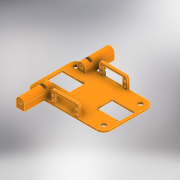
# Autodesk Inventor part: Base
Saved by Autodesk Inventor 2021 (Build 250183000, 183)
## iProperties
Created: 2024-04-05
Part Number: Base
Material: PLA
Document SubType Name: Modeling
Designer: Martin
Density: 1.27 g/cm^3
Appearance: PLA
Mass: 116.332 g
Surface Area: 562.833 cm^2
Volume: 116.332 cm^3
Author: Martin
Autodesk Inventor part; units mm, degrees
ref_plane "YZ Plane" through (0, 0, 0) normal (1, 0, 0) x (0, 1, 0)
ref_plane "XZ Plane" through (0, 0, 0) normal (0, 1, 0) x (-1, 0, 0)
sketch "Sketch1" plane through (0, 0, 0) normal (0, 0, 1) x (1, 0, 0)
  line L0 (-20.5, 0.0342) -> (20.5, 0.0342)
  line L1 (20.5, 0.0342) -> (20.5, 21.0342)
  line L2 (20.5, 21.0342) -> (-20.5, 21.0342)
  line L3 (-20.5, 21.0342) -> (-20.5, 0.0342)
  line L4 (0, -10.9658) -> (0, 38.0342) projected
  line L5 (20.5, 0.0342) -> (27.5, 0.0342)
  line L6 (20.5, 18.3469) -> (20.5, 0.0342)
  line L7 (20.5, 1.1342) -> (27.5, 1.1342)
  line L8 (27.5, 1.1342) -> (27.5, 19.9342)
  line L9 (27.5, 19.9342) -> (20.5, 19.9342)
  line L10 (20.5, 19.9342) -> (20.5, 1.1342)
  circle A0 centre (25.8, 15.5342) radius 2.3
  circle A1 centre (25.8, 5.5342) radius 2.3
  line L11 (-20.5, 0.0342) -> (-27.5, 0.0342)
  line L12 (-20.5, 1.1342) -> (-27.5, 1.1342)
  line L13 (-27.5, 19.9342) -> (-20.5, 19.9342)
  circle A2 centre (-25.8, 15.5342) radius 2.3
  circle A3 centre (-25.8, 5.5342) radius 2.3
  line L14 (-30.5, 0.0342) -> (-30.5, 31.0342)
  line L15 (30.5, 31.0342) -> (30.5, 0.0342)
  line L16 (-30.5, 26.0342) -> (30.5, 26.0342)
  line L17 (-27.5, 1.1342) -> (-27.5, 13.985)
  line L18 (-27.5, 17.0834) -> (-27.5, 19.9342)
  line L19 (-20.5, 8.5342) -> (-22.5, 8.5342)
  line L20 (-22.5, 8.5342) -> (-22.5, 12.5342)
  line L21 (-22.5, 12.5342) -> (-20.5, 12.5342)
  line L22 (-20.5, 9.5596) -> (-20.5, 7.5596)
  line L23 (-21.9602, 10.5342) -> (-18.6691, 10.5342)
  line L24 (-30.5, 0.0342) -> (-26.5, 0.0342)
  line L25 (-30.5, 0.0342) -> (30.5, 0.0342)
  line L26 (30.5, 0.0342) -> (30.5, -3.9658)
  line L27 (30.5, -3.9658) -> (-30.5, -3.9658)
  line L28 (-30.5, -3.9658) -> (-30.5, 0.0342)
  point P0 (0, 0)
  point P1 (30.5, 0.0342)
  dimension "d0" = 41
  dimension "d4" = 7
  dimension "d5" = 18.8
  dimension "d6" = 1.1
  dimension "d7" = 21
  dimension "d8" = 4.6
  dimension "d9" = 4.6
  dimension "d10" = 5.3
  dimension "d11" = 10
  dimension "d12" = 4.4
  dimension "d13" = 4.4
  dimension "d14" = 10
  dimension "d15" = 5
  dimension "d16" = 2
  dimension "d17" = 4
  dimension "d19" = 4
  constraints: 56 end point, 9 parallel, 7 horizontal, 7 symmetric about line, 4 centre point, 4 perpendicular, 3 point on line, 2 point on circle, 1 vertical alignment, 4 other
  measures "d0" distance of L0.start L0.end
  measures "d4" distance of L9.end L8.end
  measures "d5" distance of L8.end L7.end
  measures "d6" distance between parallel lines of L5 L7
  measures "d7" distance of L2.end L0.start
  measures "d8" diameter of A0
  measures "d9" diameter of A1
  measures "d10" distance from line of L6 A1.centre
  measures "d11" distance of A0.centre A1.centre
  measures "d12" distance from line of L9 A0.centre
  measures "d13" distance from line of L7 A1.centre
  measures "d14" distance between parallel lines of L3 L14
  measures "d15" distance between parallel lines of L2 L16
  measures "d16" distance of L20.end L21.end
  measures "d17" distance of L19.end L20.end
  measures "d19" distance of L25.end L26.end
extrude "Extrusion1" add sketch "Sketch1" along normal blind 5 contours L11 L24 L14 L16 L4 L2 L3 L13 L18 A2 L17 A3 L12 | L0 L4 L27 L28 L24 L11 | L0 L5 L25 L26 L27 L4 | L12 L17 A3 A2 L18 L13 L3 L21 L20 L19 | L1 L7 L8 A1 A0 L9 L2 L4 L16 L15 L25 L5 | L1 L9 L8 A0 A1 L7
sketch "Sketch2" plane through (0, 0, 5) normal (0, 0, 1) x (1, 0, 0)
  line L0 (20.5, 0.0342) -> (-20.5, 0.0342) projected
  line L1 (20.5, 0.0342) -> (12.9, 0.0342)
  line L2 (12.9, 0.0342) -> (12.9, 10.0342)
  line L3 (12.9, 10.0342) -> (-54.1, 10.0342)
  circle A0 centre (-54.1, 10.0342) radius 4.1
  circle A1 centre (-54.1, 10.0342) radius 9.1
  line L4 (-63.2, 10.0342) -> (-63.2, 0.0342)
  line L5 (-45, 10.0342) -> (-45, 0.0342)
  line L6 (-63.2, 0.0342) -> (-45, 0.0342)
  line L7 (-63.2, 0.0342) -> (-45, 0.0342)
  line L8 (-45, 0.0342) -> (-45, -3.9658)
  line L9 (-45, -3.9658) -> (-63.2, -3.9658)
  line L10 (-63.2, -3.9658) -> (-63.2, 0.0342)
  point P0 (0, 0)
  dimension "d22" = 7.6
  dimension "d23" = 10
  dimension "d24" = 67
  dimension "d25" = 8.2
  dimension "d26" = 5
  dimension "d29" = 4
  constraints: 20 end point, 3 horizontal, 2 centre point, 2 coincident, 2 parallel, 2 perpendicular, 2 point on circle, 2 point on line, 2 vertical, 1 tangent
  measures "d22" distance of L0.start L1.end
  measures "d23" distance of L1.end L2.end
  measures "d24" distance of L3.start L3.end
  measures "d25" diameter of A0
  measures "d26" radial gap between concentric circles of A0 A1
  measures "d29" distance of L7.end L8.end
extrude "Extrusion2" add sketch "Sketch2" along normal blind 43
sketch "Sketch5" plane through (0, 0, 0) normal (0, 1, 0) x (-1, 0, 0)
  line L0 (-20.5, 0) -> (-20.5, 5) projected
  line L1 (20.5, 0) -> (20.5, 5) projected
  line L2 (14.7818, 0) -> (56.1092, 0)
  line L3 (56.1092, 0) -> (56.1092, -28.5)
  line L4 (56.1092, -28.5) -> (14.7818, -28.5)
  line L5 (14.7818, -28.5) -> (14.7818, 0)
  line L6 (17.451, -24.4449) -> (17.451, -8.948) construction
  line L7 (17.451, -8.948) -> (25.6459, -8.948) construction
  line L8 (25.6459, -8.948) -> (25.6459, -24.4449) construction
  line L9 (25.6459, -24.4449) -> (17.451, -24.4449) construction
  line L10 (-84.7718, 5) -> (85.2282, 5)
  line L11 (85.2282, 5) -> (85.2282, -50)
  line L12 (85.2282, -50) -> (-84.7718, -50)
  line L13 (-84.7718, -50) -> (-84.7718, 5)
  point P0 (0, 0)
  point P1 (30.5, 5)
  dimension "d30" = 28.5
  dimension "d49" = 55
  dimension "d60" = 170
  constraints: 16 end point, 4 parallel, 2 horizontal, 2 perpendicular, 2 other
  measures "d30" distance of L2.end L3.end
  measures "d49" distance of L12.end L10.start
  measures "d60" distance of L11.end L12.end
sketch "Sketch7" plane through (0, 0, 0) normal (0, 1, 0) x (-1, 0, 0)
  point P0 (0, 0)
sketch "Sketch8" plane through (0, 0, 5) normal (0, 0, -1) x (-1, 0, 0)
  line L0 (63.2, 10.0342) -> (63.2, -3.9658) projected
  arc A0 (63.2, 10.0342) -> (45, 10.0342) centre (54.1, 10.0342) ccw projected
  line L1 (45, -3.9658) -> (45, 10.0342) projected
  line L2 (63.2, -3.9658) -> (45, -3.9658) projected
  circle A1 centre (54.1, 10.0342) radius 4.1 projected
  line L3 (63.2, 10.0342) -> (63.2, -3.9658) projected
  line L4 (63.2, 0) -> (45, 0)
  point P0 (0, 0)
  constraints: 2 end point, 2 point on line, 1 perpendicular
extrude "Extrusion4" add sketch "Sketch8" along normal blind 20 contours L0 L4 L1 A0
extrude "Extrusion5" add sketch "Sketch5" against normal blind 4 contours L10 L11 L12 L13 | L2 L3 L4 L5
ref_plane "Work Plane1" through (0, 0, 0) normal (0, 0, -1) x (-1, 0, 0)
sketch "Sketch9" plane through (0, 0, 0) normal (0, 0, -1) x (-1, 0, 0)
  line L0 (45, 10.0342) -> (45, 0) projected
  line L1 (45, 0) -> (63.2, 0) projected
  line L2 (63.2, 0) -> (63.2, 10.0342) projected
  arc A0 (63.2, 10.0342) -> (45, 10.0342) centre (54.1, 10.0342) ccw projected
  circle A1 centre (54.1, 10.0342) radius 4.1 projected
  line L3 (61.6056, 10.0342) -> (57.8528, 3.5342)
  line L4 (57.8528, 3.5342) -> (50.3472, 3.5342)
  line L5 (50.3472, 3.5342) -> (46.5944, 10.0342)
  line L6 (46.5944, 10.0342) -> (50.3472, 16.5342)
  line L7 (50.3472, 16.5342) -> (57.8528, 16.5342)
  line L8 (57.8528, 16.5342) -> (61.6056, 10.0342)
  line L9 (46.5944, 10.0342) -> (46.5944, 15.1797)
  arc A2 (63.2, 10.0342) -> (45, 10.0342) centre (54.1, 10.0342) ccw projected
  line L10 (61.6056, 10.0342) -> (61.6056, 15.1797)
  point P0 (0, 0)
  dimension "d43" = 13
  constraints: 16 end point, 2 point on circle, 2 vertical, 1 coincident, 13 other
  measures "d43" distance between parallel lines of L7 L4
extrude "Extrusion6" cut sketch "Sketch9" along normal mid plane 6.5 contours A0 L10 L8 L7 L6 L9 | L6 L7 L8 L3 L4 L5
fillet "Fillet2" radius 15 2 edges at (84.7718, -2, 5) (-85.2282, -2, 5)
fillet "Fillet3" radius 5 2 edges at (30.5, 26.0342, 2.5) (-30.5, 26.0342, 2.5)
sketch "Sketch10" plane through (0, 0, 0) normal (0, 1, 0) x (1, 0, 0)
  arc A0 (-85.2282, 10) -> (-70.2282, -5) centre (-70.2282, 10) ccw projected
  line L0 (-63.2, -5) -> (-63.2, 15) projected
  line L1 (-45, 15) -> (-63.2, 15) projected
  line L2 (-45, -5) -> (-45, 15) projected
  line L3 (-45, -5) -> (-30.5, -5) projected
  line L4 (-30.5, 0) -> (-30.5, -5) projected
  line L5 (30.5, 0) -> (-30.5, 0) projected
  line L6 (30.5, -5) -> (30.5, 0) projected
  line L7 (30.5, -5) -> (69.7718, -5) projected
  arc A1 (69.7718, -5) -> (84.7718, 10) centre (69.7718, 10) ccw projected
  line L8 (84.7718, 10) -> (84.7718, 50) projected
  line L9 (84.7718, 50) -> (-85.2282, 50) projected
  line L10 (-85.2282, 50) -> (-85.2282, 10) projected
  line L11 (-70.2282, -5) -> (-63.2, -5) projected
  point P0 (0, 0)
  constraints: 2 coincident
hole "Hole1" at (-70.2282, 0, -10) at (69.7718, 0, -10) direction (0, -1, 0) diameter 10 depth 4
mirror "Mirror4" about plane through (-85.2282, 0, -50) normal (0, 0, -1) of "Extrusion1", "Extrusion2", "Extrusion4", "Extrusion5", "Extrusion6", "Fillet2", "Fillet3", "Hole1"
sketch "Sketch11" plane through (0, 0, 0) normal (0, 1, 0) x (1, 0, 0)
  circle A0 centre (69.7718, 90) radius 5 projected
  circle A1 centre (69.7718, 10) radius 5 projected
  arc A2 (-70.2282, 105) -> (-85.2282, 90) centre (-70.2282, 90) ccw projected
  line L0 (-85.2282, 90) -> (-85.2282, 10) projected
  arc A3 (-85.2282, 10) -> (-70.2282, -5) centre (-70.2282, 10) ccw projected
  line L1 (-63.2, -5) -> (-63.2, 15) projected
  line L2 (-45, 15) -> (-63.2, 15) projected
  line L3 (-45, -5) -> (-45, 15) projected
  line L4 (-45, -5) -> (-30.5, -5) projected
  line L5 (-30.5, 0) -> (-30.5, -5) projected
  line L6 (30.5, 0) -> (-30.5, 0) projected
  line L7 (30.5, -5) -> (30.5, 0) projected
  line L8 (30.5, -5) -> (69.7718, -5) projected
  arc A4 (69.7718, -5) -> (84.7718, 10) centre (69.7718, 10) ccw projected
  line L9 (84.7718, 10) -> (84.7718, 90) projected
  arc A5 (84.7718, 90) -> (69.7718, 105) centre (69.7718, 90) ccw projected
  line L10 (30.5, 105) -> (69.7718, 105) projected
  line L11 (30.5, 105) -> (30.5, 100) projected
  line L12 (30.5, 100) -> (-30.5, 100) projected
  line L13 (-30.5, 100) -> (-30.5, 105) projected
  line L14 (-45, 105) -> (-30.5, 105) projected
  line L15 (-45, 105) -> (-45, 85) projected
  line L16 (-45, 85) -> (-63.2, 85) projected
  line L17 (-63.2, 105) -> (-63.2, 85) projected
  line L18 (20.5, 100) -> (-20.5, 100) projected
  line L19 (20.5, 100) -> (20.5, 105) projected
  line L20 (20.5, 105) -> (-20.5, 105) projected
  line L21 (-20.5, 100) -> (-20.5, 105) projected
  line L22 (-20.5, 100) -> (20.5, 100)
  line L23 (20.5, 100) -> (20.5, 71.5)
  line L24 (20.5, 71.5) -> (-20.5, 71.5)
  line L25 (-20.5, 71.5) -> (-20.5, 100)
  line L26 (74.1747, 78.4479) -> (24.1747, 78.4479)
  line L27 (24.1747, 78.4479) -> (24.1747, 28.4479)
  line L28 (24.1747, 28.4479) -> (74.1747, 28.4479)
  line L29 (74.1747, 28.4479) -> (74.1747, 78.4479)
  line L30 (0, 73.183) -> (0, 43.8378)
  line L31 (-78.2096, 79.1815) -> (-28.2096, 79.1815)
  line L32 (-28.2096, 79.1815) -> (-28.2096, 29.1815)
  line L33 (-28.2096, 29.1815) -> (-78.2096, 29.1815)
  line L34 (-78.2096, 29.1815) -> (-78.2096, 79.1815)
  circle A6 centre (-70.2282, 90) radius 5 projected
  line L35 (-70.2282, 105) -> (-63.2, 105) projected
  line L36 (-70.2282, -5) -> (-63.2, -5) projected
  circle A7 centre (-70.2282, 10) radius 5 projected
  point P0 (0, 0)
  dimension "d57" = 28.5
  dimension "d58" = 50
  dimension "d59" = 50
  constraints: 26 end point, 4 parallel, 2 horizontal, 2 perpendicular, 1 vertical
  measures "d57" distance of L22.end L23.end
  measures "d58" distance of L28.end L27.end
  measures "d59" distance of L27.end L26.end
sketch "Sketch12" plane through (0, 0, 0) normal (0, 1, 0) x (1, 0, 0)
  line L0 (-79.2036, 26.0949) -> (-29.2036, 26.0949)
  line L1 (-29.2036, 26.0949) -> (-29.2036, 76.0949)
  line L2 (-29.2036, 76.0949) -> (-79.2036, 76.0949)
  line L3 (-79.2036, 76.0949) -> (-79.2036, 26.0949)
  circle A0 centre (-74.6036, 31.6949) radius 1.6
  line L4 (-85.2282, 90) -> (-85.2282, 10) projected
  circle A1 centre (-33.8036, 32.0949) radius 1.6
  circle A2 centre (-34.2036, 70.4949) radius 1.6
  line L5 (-79.2036, 34.2067) -> (-29.2036, 34.2067)
  line L6 (-29.2036, 34.2067) -> (-29.2036, 68.2067)
  line L7 (-29.2036, 68.2067) -> (-79.2036, 68.2067)
  line L8 (-79.2036, 68.2067) -> (-79.2036, 34.2067)
  circle A3 centre (-73.0036, 70.4949) radius 1.6
  line L9 (29.7223, 26.0949) -> (79.7223, 26.0949)
  line L10 (79.7223, 26.0949) -> (79.7223, 76.0949)
  line L11 (79.7223, 76.0949) -> (29.7223, 76.0949)
  line L12 (29.7223, 76.0949) -> (29.7223, 26.0949)
  circle A4 centre (34.3223, 31.6949) radius 1.6
  circle A5 centre (75.1223, 32.0949) radius 1.6
  circle A6 centre (74.7223, 70.4949) radius 1.6
  line L13 (29.7223, 34.2067) -> (79.7223, 34.2067)
  line L14 (79.7223, 34.2067) -> (79.7223, 68.2067)
  line L15 (79.7223, 68.2067) -> (29.7223, 68.2067)
  line L16 (29.7223, 68.2067) -> (29.7223, 34.2067)
  circle A7 centre (35.9223, 70.4949) radius 1.6
  point P0 (0, 0)
  dimension "d67" = 50
  dimension "d68" = 50
  dimension "d69" = 3.2
  dimension "d70" = 4.6
  dimension "d71" = 10.6246
  dimension "d72" = 5.6
  dimension "d73" = 3.2
  dimension "d74" = 4.6
  dimension "d75" = 3.2
  dimension "d76" = 5.6
  dimension "d88" = 34
  dimension "d89" = 3.2
  dimension "d90" = 50
  dimension "d91" = 50
  dimension "d92" = 3.2
  dimension "d93" = 4.6
  dimension "d94" = 5.6
  dimension "d95" = 3.2
  dimension "d96" = 4.6
  dimension "d97" = 3.2
  dimension "d98" = 5.6
  dimension "d99" = 34
  dimension "d100" = 3.2
  constraints: 32 end point, 8 centre point, 8 parallel, 4 horizontal, 4 perpendicular, 4 point on line
  measures "d67" distance of L2.end L1.end
  measures "d68" distance of L1.end L0.end
  measures "d69" diameter of A0
  measures "d70" distance from line of L3 A0.centre
  measures "d71" distance from line of A0.centre L4
  measures "d72" distance from line of L0 A0.centre
  measures "d73" diameter of A1
  measures "d74" distance from line of L1 A1.centre
  measures "d75" diameter of A2
  measures "d76" distance from line of L2 A2.centre
  measures "d88" distance of L6.end L5.end
  measures "d89" diameter of A3
  measures "d90" distance of L12.start L11.start
  measures "d91" distance of L11.start L9.end
  measures "d92" diameter of A4
  measures "d93" distance from line of L12 A4.centre
  measures "d94" distance from line of L9 A4.centre
  measures "d95" diameter of A5
  measures "d96" distance from line of L10 A5.centre
  measures "d97" diameter of A6
  measures "d98" distance from line of L11 A6.centre
  measures "d99" distance of L15.start L13.end
  measures "d100" diameter of A7
extrude "Extrusion7" cut sketch "Sketch12" against normal up to next contours L3 L7 L1 L5 | A0 | A1 | A2 | A3 | L12 L15 L10 L13 | A4 | A5 | A6 | A7
equation "\"d6\" = -0.5 * d5 + 0.5 * d7"
equation "\"d12\" = d13"
equation "\"d73\" = d69"
equation "\"d74\" = d70"
equation "\"d75\" = d69"
equation "\"d76\" = d72"
equation "\"d89\" = d69"
equation "\"d95\" = d92"
equation "\"d96\" = d93"
equation "\"d97\" = d92"
equation "\"d98\" = d94"
equation "\"d100\" = d92"
body "Solid1"
